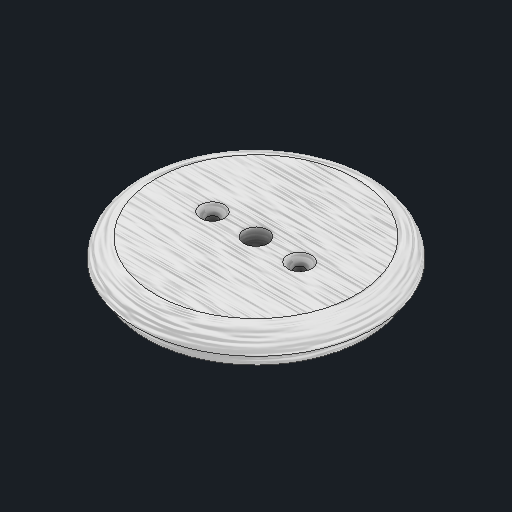
# Autodesk Inventor part: Tapa
Saved by Autodesk Inventor 2025.3 (Build 293356030, 356C)
## iProperties
Created: 2024-12-23
Part Number: Tapa
Material: Aluminum 7075
Document SubType Name: Modeling
Designer: Usuario
Density: 2.81 g/cm^3
Appearance: Satin - Brushed Heavy
Mass: 96.7212 g
Surface Area: 197.809 cm^2
Volume: 96.7212 cm^3
Author: Usuario
Autodesk Inventor part; units mm, degrees
ref_plane "YZ Plane" through (0, 0, 0) normal (1, 0, 0) x (0, 1, 0)
ref_plane "XZ Plane" through (0, 0, 0) normal (0, 1, 0) x (-1, 0, 0)
ref_plane "XY Plane" through (0, 0, 0) normal (0, 0, 1) x (1, 0, 0)
sketch "Boceto1" plane through (0, 0, 0) normal (0, 1, 0) x (-1, 0, 0)
  circle A0 centre (0, 0) radius 50
  dimension "Diametro" = 100
  constraints: 1 centre point, 1 coincident
  measures "Diametro" diameter of A0
extrude "Extrusión1" add sketch "Boceto1" against normal blind 8
fillet "Empalme1" radius 8 1 edges at (50, 0, 0)
sketch "Boceto2" plane through (0, -8, 0) normal (0, -1, 0) x (1, 0, 0)
  circle A0 centre (0, 0) radius 46
  circle A1 centre (0, 0) radius 50 projected
  dimension "d22" = 4
  constraints: 1 centre point, 1 coincident
  measures "d22" radial gap between concentric circles of A1 A0
extrude "Extrusión3" add sketch "Boceto2" along normal blind 6 contours A0
sketch "Boceto3" plane through (0, -14, 0) normal (0, -1, 0) x (1, 0, 0)
  point P0 (0, 0)
  point P1 (-37.5, 0)
  point P2 (-18.75, -32.476)
  point P3 (18.75, -32.476)
  point P4 (37.5, 0)
  point P5 (18.75, 32.476)
  point P6 (-18.75, 32.476)
  dimension "d25" = 37.5
  dimension "d35" = 360
  constraints: 1 horizontal alignment, 7 other
  measures "d25" distance of point (0, 0) point (-37.5, 0)
hole "Agujero2" at (-37.5, -14, 0) at (-18.75, -14, 32.476) at (-18.75, -14, -32.476) at (18.75, -14, 32.476) at (37.5, -14, 0) at (18.75, -14, -32.476) direction (0, 1, 0) diameter 2.459 depth 8.8 thread size "M3x0.5" class "6H" standard "ANSI Metric M Profile"
sketch "Boceto4" plane through (0, -14, 0) normal (0, -1, 0) x (1, 0, 0)
  arc A0 (20.5788, -4.4246) -> (20.5788, 4.4246) centre (18.25, 0) ccw
  line L0 (20.5788, 4.4246) -> (6.2877, 11.9463)
  arc A1 (6.2877, 11.9463) -> (-6.2877, 11.9463) centre (0, 0) ccw
  line L1 (-6.2877, 11.9463) -> (-20.5788, 4.4246)
  arc A2 (-20.5788, 4.4246) -> (-20.5788, -4.4246) centre (-18.25, 0) ccw
  line L2 (-20.5788, -4.4246) -> (-6.2877, -11.9463)
  arc A3 (-6.2877, -11.9463) -> (6.2877, -11.9463) centre (0, 0) ccw
  line L3 (6.2877, -11.9463) -> (20.5788, -4.4246)
  line L4 (-17.0094, 4.3256) -> (-5.4726, 10.3977)
  arc A4 (5.4726, 10.3977) -> (-5.4726, 10.3977) centre (0, 0) ccw
  line L5 (5.4726, 10.3977) -> (17.0094, 4.3256)
  arc A5 (17.0094, 4.3256) -> (17.0094, -4.3256) centre (18.25, 0) ccw
  line L6 (17.0094, -4.3256) -> (5.4726, -10.3977)
  arc A6 (-5.4726, -10.3977) -> (5.4726, -10.3977) centre (0, 0) ccw
  line L7 (-5.4726, -10.3977) -> (-17.0094, -4.3256)
  arc A7 (-17.0094, -4.3256) -> (-17.0094, 4.3256) centre (-18.25, 0) ccw
  circle A8 centre (18.25, 0) radius 2.5
  circle A9 centre (-18.25, 0) radius 2.5
  point P0 (0, 0)
  point P1 (20.5788, 4.4246)
  point P2 (-6.2877, 11.9463)
  point P3 (-20.5788, -4.4246)
  point P4 (6.2877, -11.9463)
  dimension "d3" = 8
  constraints: 16 end point, 16 point on circle, 10 centre point, 61 other
extrude "Extrusión5" cut sketch "Boceto4" against normal blind 4 contours L3 A3 L2 A2 L1 A1 L0 A0 | L4 A4 L5 A5 L6 A6 L7 A7 | A8 | A9
sketch "Boceto5" plane through (0, -14, 0) normal (0, -1, 0) x (1, 0, 0)
  line L0 (6.2877, 11.9463) -> (20.5788, 4.4246) projected
  arc A0 (6.2877, 11.9463) -> (-6.2877, 11.9463) centre (0, 0) ccw projected
  line L1 (-20.5788, 4.4246) -> (-6.2877, 11.9463) projected
  arc A1 (-20.5788, 4.4246) -> (-20.5788, -4.4246) centre (-18.25, 0) ccw projected
  line L2 (-6.2877, -11.9463) -> (-20.5788, -4.4246) projected
  arc A2 (-6.2877, -11.9463) -> (6.2877, -11.9463) centre (0, 0) ccw projected
  line L3 (20.5788, -4.4246) -> (6.2877, -11.9463) projected
  arc A3 (20.5788, -4.4246) -> (20.5788, 4.4246) centre (18.25, 0) ccw projected
  arc A4 (6.4041, 12.1676) -> (-6.4041, 12.1676) centre (0, 0) ccw
  line L4 (6.4041, 12.1676) -> (20.6952, 4.6458)
  arc A5 (20.6952, -4.6458) -> (20.6952, 4.6458) centre (18.25, 0) ccw
  line L5 (20.6952, -4.6458) -> (6.4041, -12.1676)
  arc A6 (-6.4041, -12.1676) -> (6.4041, -12.1676) centre (0, 0) ccw
  line L6 (-6.4041, -12.1676) -> (-20.6952, -4.6458)
  arc A7 (-20.6952, 4.6458) -> (-20.6952, -4.6458) centre (-18.25, 0) ccw
  line L7 (-20.6952, 4.6458) -> (-6.4041, 12.1676)
  point P0 (0, 0)
  dimension "d44" = 0.25
  constraints: 8 end point, 8 point on circle, 4 centre point, 7 other
  measures "d44" distance between parallel lines of L1 L7
extrude "Extrusión7" cut sketch "Boceto5" against normal up to surface (4 mm away) contours L0 A3 L3 A2 L2 A1 L1 A0 | L4 A5 L5 A6 L6 A7 L7 A4
sketch "Boceto6" plane through (0, 0, 0) normal (0, 1, 0) x (1, 0, 0)
  point P0 (0, 0)
  point P1 (-18.25, 0)
  point P2 (18.25, 0)
hole "Agujero3" at (-18.25, 0, 0) at (18.25, 0, 0) direction (0, -1, 0) diameter 4.134 end through all countersink diameter 10 countersink angle 90 thread size "M5x0.8" class "6H" standard "ISO Metric profile"
sketch "Boceto7" plane through (0, 0, 0) normal (0, 1, 0) x (1, 0, 0)
  circle A0 centre (0, 0) radius 5
  dimension "d54" = 10
  constraints: 1 centre point, 1 coincident
  measures "d54" diameter of A0
extrude "Extrusión8" cut sketch "Boceto7" against normal through all
sketch "Boceto9" plane through (0, 0, 0) normal (0, 1, 0) x (1, 0, 0)
  circle A0 centre (0, 0) radius 8.0135
  circle A1 centre (0, 0) radius 5
  dimension "d57" = 16.027
  dimension "d58" = 10
  constraints: 2 centre point, 2 coincident
  measures "d57" diameter of A0
  measures "d58" diameter of A1
extrude "Extrusión9" [suppressed]
extrude "Extrusión10" [suppressed]
